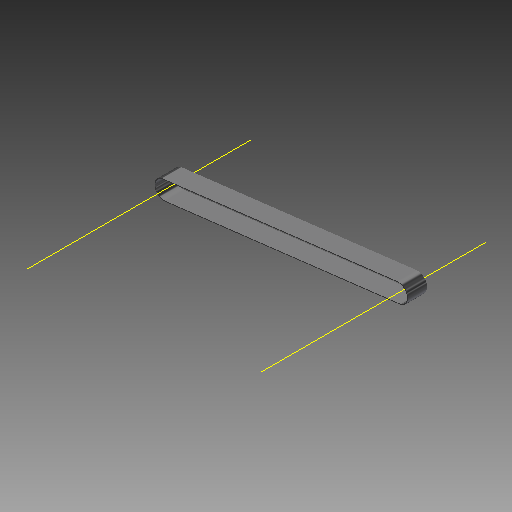
# Autodesk Inventor part: Synchronous Belt
Saved by Autodesk Inventor 2019.4 (Build 234330000, 330)
## iProperties
Created: 2020-01-11
Part Number: Synchronous Belt
Material: Rubber
Document SubType Name: Modeling
Designer: admin
Density: 0.93 g/cm^3
Appearance: Rubber - Black - Version 1.1
Mass: 16.0425 g
Surface Area: 358.8 cm^2
Volume: 17.25 cm^3
CustomPartVersion: 1
Author: admin
Autodesk Inventor part; units mm, degrees
sketch "Sketch Path" plane through (0, 0, 0) normal (0, 0, 1) x (1, 0, 0)
  arc A0 (-52.314023, -185.869602) -> (-55.172713, -162.168135) centre (-53.743368, -174.018868) ccw
  arc A1 (-360.46017, -198.989577) -> (-357.60148, -222.691044) centre (-359.030825, -210.84031) ccw
  line L0 (-360.46017, -198.989577) -> (-55.172713, -162.168135)
  line L1 (-52.314023, -185.869602) -> (-357.60148, -222.691044)
  constraints: 4 end point, 4 point on circle, 2 centre point
ref_plane "Cross Section Plane" through (-55.172713, -162.168135, 0) normal (-0.9928047, -0.1197445, 0) x (0, 0, 1)
ref_plane "Work Plane2" through (-53.743368, -174.018868, 0) normal (-1, 0, 0) x (0, 0, 1)
ref_plane "Work Plane3" through (-359.030825, -210.84031, 0) normal (1, 0, 0) x (0, 0, 1)
sketch "Cross Section" plane through (-55.172713, -162.168135, 0) normal (-0.9928047, -0.1197445, 0) x (0, 0, 1)
  line L0 (-12.5, 0.5) -> (12.5, 0.5)
  line L1 (12.5, 0.5) -> (12.5, -0.5)
  line L2 (12.5, -0.5) -> (-12.5, -0.5)
  line L3 (-12.5, -0.5) -> (-12.5, 0.5)
  line L4 (-12.5, 0) -> (12.5, 0) construction
  point P0 (0, 0)
  point P1 (0, 0)
  dimension "d0" = 25
  dimension "d4" = 0.5
  dimension "d5" = 0.5
  constraints: 10 end point, 3 midpoint, 2 parallel, 1 coincident, 1 horizontal, 1 perpendicular, 1 other
  measures "d0" distance between parallel lines of L1 L3
  measures "d4" distance between parallel lines of L2 L4
  measures "d5" distance between parallel lines of L4 L0
sweep "Belt" add profiles "Cross Section" path "Sketch Path" path curves L1 A1 L0 A0
equation "\"d0\" = da_B"
equation "\"d4\" = da_a"
equation "\"d5\" = da_a2"
equation "\"da_B\" = 25"
equation "\"da_pb\" = 5"
equation "\"da_a\" = 0.5"
equation "\"da_S\" = 2.65"
equation "\"da_Beta\" = 20deg"
equation "\"da_Ht\" = 1.2"
equation "\"da_H\" = 2.2"
equation "\"da_a2\" = 0.5"
body "Solid1"
